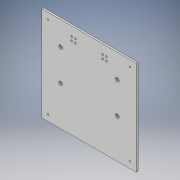
# Autodesk Inventor part: base_plate_v1
Saved by Autodesk Inventor 2019 (Build 230136000, 136)
## iProperties
Created: 2018-09-28
Part Number: base_plate_v1
Material: Generic
Document SubType Name: Modeling
Designer: Brian
Density: 1 g/cm^3
Appearance: Default
Author: Brian
Autodesk Inventor part; units mm, degrees
ref_plane "YZ Plane" through (0, 0, 0) normal (1, 0, 0) x (0, 1, 0)
ref_plane "XZ Plane" through (0, 0, 0) normal (0, 1, 0) x (-1, 0, 0)
ref_plane "XY Plane" through (0, 0, 0) normal (0, 0, 1) x (1, 0, 0)
sketch "Sketch1" plane through (0, 0, 0) normal (0, 0, 1) x (1, 0, 0)
  line L0 (0, 0) -> (300, 0)
  line L1 (300, 0) -> (300, 300)
  line L2 (300, 300) -> (0, 300)
  line L3 (0, 300) -> (0, 0)
  dimension "d0" = 300
  dimension "d1" = 300
  constraints: 8 end point, 2 parallel, 1 horizontal, 1 perpendicular
  measures "d0" distance of L2.end L1.end
  measures "d1" distance of L1.end L0.end
extrude "Extrusion1" add sketch "Sketch1" along normal blind 6
sketch "Sketch2" plane through (0, 0, 6) normal (0, 0, 1) x (1, 0, 0)
  line L0 (300, 0) -> (300, 300) projected
  line L1 (300, 300) -> (0, 300) projected
  point P0 (0, 0)
  point P1 (280, 280)
  dimension "d32" = 20
  dimension "d33" = 20
  measures "d32" distance from line of L0 point (280, 280)
  measures "d33" distance from line of L1 point (280, 280)
hole "Hole1" at (280, 280, 6) direction (0, 0, -1) diameter 5 end through all
sketch "Sketch3" plane through (0, 0, 6) normal (0, 0, 1) x (1, 0, 0)
  line L0 (0, 300) -> (0, 0) projected
  line L1 (300, 300) -> (0, 300) projected
  point P0 (20, 280)
  dimension "d34" = 20
  dimension "d35" = 20
  measures "d34" distance from line of L0 point (20, 280)
  measures "d35" distance from line of L1 point (20, 280)
hole "Hole2" at (20, 280, 6) direction (0, 0, -1) diameter 5 end through all
sketch "Sketch4" plane through (0, 0, 6) normal (0, 0, 1) x (1, 0, 0)
  line L0 (0, 0) -> (300, 0) projected
  line L1 (0, 300) -> (0, 0) projected
  point P0 (20, 20)
  dimension "d36" = 20
  dimension "d37" = 20
  measures "d36" distance from line of L0 point (20, 20)
  measures "d37" distance from line of L1 point (20, 20)
hole "Hole3" at (20, 20, 6) direction (0, 0, -1) diameter 5 end through all
sketch "Sketch5" plane through (0, 0, 6) normal (0, 0, 1) x (1, 0, 0)
  line L0 (0, 0) -> (300, 0) projected
  line L1 (300, 0) -> (300, 300) projected
  point P0 (280, 20)
  dimension "d38" = 20
  dimension "d39" = 20
  measures "d38" distance from line of L0 point (280, 20)
  measures "d39" distance from line of L1 point (280, 20)
hole "Hole4" at (280, 20, 6) direction (0, 0, -1) diameter 5 end through all
sketch "Sketch6" plane through (0, 0, 6) normal (0, 0, 1) x (1, 0, 0)
  line L0 (300, 300) -> (0, 300) projected
  line L1 (300, 0) -> (300, 300) projected
  point P0 (0, 0)
  point P1 (240, 225)
  dimension "d68" = 75
  dimension "d69" = 60
  measures "d68" distance from line of L0 point (240, 225)
  measures "d69" distance from line of L1 point (240, 225)
hole "Hole5" at (240, 225, 6) direction (0, 0, -1) diameter 12 end through all
sketch "Sketch7" plane through (0, 0, 6) normal (0, 0, 1) x (1, 0, 0)
  line L0 (300, 0) -> (300, 300) projected
  circle A0 centre (240, 225) radius 6 projected
  point P0 (0, 0)
  point P1 (240, 125)
  dimension "d72" = 60
  dimension "d73" = 100
  measures "d72" distance from line of L0 point (240, 125)
  measures "d73" distance of A0.centre point (240, 125)
hole "Hole6" at (240, 125, 6) direction (0, 0, -1) diameter 12 end through all
sketch "Sketch8" plane through (0, 0, 6) normal (0, 0, 1) x (1, 0, 0)
  line L0 (300, 300) -> (0, 300) projected
  line L1 (0, 300) -> (0, 0) projected
  point P0 (60, 225)
  dimension "d70" = 75
  dimension "d71" = 60
  measures "d70" distance from line of L0 point (60, 225)
  measures "d71" distance from line of L1 point (60, 225)
hole "Hole7" at (60, 225, 6) direction (0, 0, -1) diameter 12 end through all
sketch "Sketch9" plane through (0, 0, 6) normal (0, 0, 1) x (1, 0, 0)
  line L0 (0, 300) -> (0, 0) projected
  circle A0 centre (60, 225) radius 6 projected
  point P0 (60, 125)
  dimension "d74" = 60
  dimension "d75" = 100
  measures "d74" distance from line of L0 point (60, 125)
  measures "d75" distance of A0.centre point (60, 125)
hole "Hole8" at (60, 125, 6) direction (0, 0, -1) diameter 12 end through all
sketch "Sketch10" plane through (0, 0, 6) normal (0, 0, 1) x (1, 0, 0)
  line L0 (300, 300) -> (0, 300) projected
  line L1 (300, 0) -> (300, 300) projected
  line L2 (0, 300) -> (0, 0) projected
  point P0 (193.3, 271)
  point P1 (205.3, 271)
  point P2 (193.3, 259)
  point P3 (205.3, 259)
  point P4 (94.8, 271)
  point P5 (106.8, 271)
  point P6 (94.8, 259)
  point P7 (106.8, 259)
  dimension "d83" = 29
  dimension "d84" = 29
  dimension "d85" = 29
  dimension "d86" = 29
  dimension "d87" = 12
  dimension "d88" = 12
  dimension "d89" = 12
  dimension "d90" = 12
  dimension "d91" = 12
  dimension "d92" = 12
  dimension "d93" = 12
  dimension "d94" = 12
  dimension "d97" = 106.7
  dimension "d98" = 106.7
  dimension "d101" = 86.5
  dimension "d102" = 86.5
  measures "d83" distance from line of L0 point (205.3, 271)
  measures "d84" distance from line of L0 point (193.3, 271)
  measures "d85" distance from line of L0 point (106.8, 271)
  measures "d86" distance from line of L0 point (94.8, 271)
  measures "d87" distance of point (205.3, 271) point (205.3, 259)
  measures "d88" distance of point (193.3, 271) point (193.3, 259)
  measures "d89" distance of point (205.3, 259) point (193.3, 259)
  measures "d90" distance of point (205.3, 271) point (193.3, 271)
  measures "d91" distance of point (106.8, 271) point (94.8, 271)
  measures "d92" distance of point (106.8, 259) point (94.8, 259)
  measures "d93" distance of point (106.8, 271) point (106.8, 259)
  measures "d94" distance of point (94.8, 271) point (94.8, 259)
  measures "d97" distance from line of L1 point (193.3, 259)
  measures "d98" distance from line of L1 point (193.3, 271)
  measures "d101" distance of point (193.3, 271) point (106.8, 271)
  measures "d102" distance of point (193.3, 259) point (106.8, 259)
hole "Hole9" at (193.3, 271, 6) at (205.3, 271, 6) at (193.3, 259, 6) at (205.3, 259, 6) at (94.8, 271, 6) at (106.8, 271, 6) at (94.8, 259, 6) at (106.8, 259, 6) direction (0, 0, -1) diameter 3.1 end through all counterbore diameter 5.7 counterbore depth 3.5
body "Solid1"
